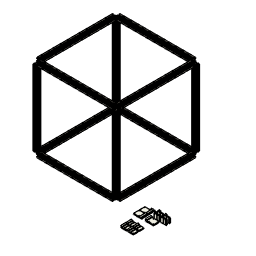
알루미늄 프로파일 20mm + 센서 케이스 v1+2+3 (Autodesk Fusion 360 design; units mm, degrees)
part number: 2025-07-09-12-54-32-083
Autodesk Fusion 360 part; units mm, degrees
note: some values were not read from the file. Set by a fixed rule: which sketch regions a step uses.
sketch "스케치1" plane through (0, 0, 0) normal (0, 0, 1) x (1, 0, 0)
  line L0 (20, 0) -> (17, 0)
  line L1 (20, 3) -> (20, 0)
  circle A0 centre (17, 3) radius 2
  circle A1 centre (17, 17) radius 2
  circle A2 centre (3, 17) radius 2
  circle A3 centre (3, 3) radius 2
  line L2 (12.65, 0) -> (12.65, 1.5)
  line L3 (12.65, 1.5) -> (14.15, 1.5)
  line L4 (14.15, 1.5) -> (14.15, 5.132)
  line L5 (7.35, 0) -> (7.35, 1.5)
  line L6 (7.35, 1.5) -> (5.85, 1.5)
  line L7 (5.85, 1.5) -> (5.85, 5.132)
  arc A4 (14.15, 5.132) -> (5.85, 5.132) centre (10, 0) ccw
  line L8 (0, 0) -> (7.35, 0)
  line L9 (12.65, 0) -> (20, 0)
  line L10 (12.65, 20) -> (12.65, 18.5)
  line L11 (12.65, 18.5) -> (14.15, 18.5)
  line L12 (14.15, 18.5) -> (14.15, 14.868)
  arc A5 (14.15, 14.868) -> (5.85, 14.868) centre (10, 20) cw
  line L13 (5.85, 18.5) -> (5.85, 14.868)
  line L14 (7.35, 18.5) -> (5.85, 18.5)
  line L15 (7.35, 20) -> (7.35, 18.5)
  line L16 (20, 12.65) -> (18.5, 12.65)
  line L17 (18.5, 12.65) -> (18.5, 14.15)
  line L18 (18.5, 14.15) -> (14.868, 14.15)
  arc A6 (14.868, 14.15) -> (14.868, 5.85) centre (20, 10) ccw
  line L19 (18.5, 5.85) -> (14.868, 5.85)
  line L20 (18.5, 7.35) -> (18.5, 5.85)
  line L21 (20, 7.35) -> (18.5, 7.35)
  line L22 (0, 7.35) -> (1.5, 7.35)
  line L23 (1.5, 7.35) -> (1.5, 5.85)
  line L24 (1.5, 5.85) -> (5.132, 5.85)
  arc A7 (5.132, 5.85) -> (5.132, 14.15) centre (0, 10) ccw
  line L25 (1.5, 14.15) -> (5.132, 14.15)
  line L26 (1.5, 12.65) -> (1.5, 14.15)
  line L27 (0, 12.65) -> (1.5, 12.65)
  line L28 (0, 20) -> (0, 12.65)
  line L29 (0, 7.35) -> (0, 0)
  line L30 (20, 0) -> (20, 7.35)
  line L31 (20, 12.65) -> (20, 20)
  line L32 (20, 20) -> (12.65, 20)
  line L33 (7.35, 20) -> (0, 20)
  line L34 (20, 12.65) -> (20, 7.35)
  dimension "d1" = 20
  dimension "d2" = 20
  dimension "d3" = 3
  dimension "d4" = 3
  dimension "d5" = 4
  dimension "d6" = 4
  dimension "d7" = 4
  dimension "d8" = 4
  dimension "d10" = 1.5
  dimension "d11" = 1.5
  dimension "d14" = 1.5
  dimension "d15" = 1.5
  dimension "d16" = 1.5
  dimension "d17" = 1.5
  dimension "d18" = 1.5
  dimension "d19" = 1.5
  dimension "d20" = 1.5
  dimension "d21" = 1.5
  dimension "d22" = 1.5
  dimension "d23" = 1.5
  dimension "d24" = 1.5
  dimension "d25" = 1.5
  dimension "d26" = 1.5
  dimension "d27" = 1.5
  constraint horizontal L8
  constraint vertical L30
  constraint horizontal L32
  constraint vertical L28
  constraint coincident L8.start L29.end
  constraint horizontal L0
  constraint vertical L1
  constraint perpendicular L2 L3
  constraint perpendicular L3 L4
  constraint perpendicular L5 L8
  constraint perpendicular L5 L6
  constraint perpendicular L6 L7
  constraint collinear L8 L9
  constraint perpendicular L10 L11
  constraint perpendicular L11 L12
  constraint perpendicular L14 L15
  constraint perpendicular L13 L14
  constraint perpendicular L16 L17
  constraint perpendicular L17 L18
  constraint perpendicular L20 L21
  constraint perpendicular L19 L20
  constraint perpendicular L22 L23
  constraint perpendicular L23 L24
  constraint perpendicular L26 L27
  constraint perpendicular L25 L26
  constraint collinear L28 L29
  constraint coincident A7.centre L28
  constraint collinear L30 L31
  constraint coincident A6.centre L30
  constraint collinear L32 L33
  constraint coincident A5.centre L32
  constraint perpendicular L21 L34
  measures "d1" distance of L8.start L0.start
  measures "d2" distance of L8.start L28.start
  measures "d3" distance of L0.start L0.end
  measures "d4" distance of L0.start L1.start
  measures "d5" diameter of A0
  measures "d6" diameter of A1
  measures "d7" diameter of A2
  measures "d8" diameter of A3
  measures "d10" distance of L2.start L2.end
  measures "d11" distance of L2.end L3.end
  measures "d14" distance of L5.start L5.end
  measures "d15" distance of L5.end L6.end
  measures "d16" distance of L10.start L10.end
  measures "d17" distance of L10.end L11.end
  measures "d18" distance of L14.start L15.start
  measures "d19" distance of L14.start L13.start
  measures "d20" distance of L16.start L16.end
  measures "d21" distance of L16.end L17.end
  measures "d22" distance of L20.start L21.start
  measures "d23" distance of L20.start L19.start
  measures "d24" distance of L22.start L22.end
  measures "d25" distance of L22.end L23.end
  measures "d26" distance of L26.start L27.start
  measures "d27" distance of L26.start L25.start
extrude "돌출1" add sketch "스케치1" along normal blind 400 contours L0 L1 L2 L3 L4 L5 L6 L7 A4 L8 L9 L10 L11 L12 A5 L13 L14 L15 L16 L17 L18 A6 L19 L20 L21 L22 L23 L24 A7 L25 L26 L27 L28 L29 L30 L31 L32 L33 | A0 | A1 | A2 | A3 makes body 1
move_body "이동1" bodies 1 to x (1, 0, 0) y (0, 0, -1) z (0, 1, 0) at (0, 0, 20)
move_body "이동2" bodies 1 to x (1, 0, 0) y (0, 1, 0) z (0, 0, 1) at (0, 20, 0)
move_body "이동3" bodies 1 to x (1, 0, 0) y (0, 1, 0) z (0, 0, 1) at (0, 5, 0)
extrude "돌출2" add sketch "스케치1" along normal blind 400 separate body contours L0 L1 L2 L3 L4 L5 L6 L7 A4 L8 L9 L10 L11 L12 A5 L13 L14 L15 L16 L17 L18 A6 L19 L20 L21 L22 L23 L24 A7 L25 L26 L27 L28 L29 L30 L31 L32 L33 makes body 2
move_body "이동4" bodies 2 to x (1, 0, 0) y (0, 1, 0) z (0, 0, 1) at (0, 0, 20)
move_body "이동5" bodies 1 to x (1, 0, 0) y (0, 1, 0) z (0, 0, 1) at (0, -5, 0)
copy_body "CopyPasteBodies1" bodies 1 makes body 3
move_body "이동6" bodies 3 to x (1, 0, 0) y (0, 1, 0) z (0, 0, 1) at (0, 0, 420)
copy_body "CopyPasteBodies2" bodies 2 makes body 4
move_body "이동7" bodies 4 to x (1, 0, 0) y (0, 1, 0) z (0, 0, 1) at (0, 420, 0)
extrude "돌출3" add sketch "스케치1" against normal blind 400 separate body contours L0 L1 L2 L3 L4 L5 L6 L7 A4 L8 L9 L10 L11 L12 A5 L13 L14 L15 L16 L17 L18 A6 L19 L20 L21 L22 L23 L24 A7 L25 L26 L27 L28 L29 L30 L31 L32 L33 makes body 5
move_body "이동8" bodies 5 to x (0, 0, 1) y (0, 1, 0) z (-1, 0, 0) at (-400, 0, 0)
copy_body "CopyPasteBodies3" bodies 5 makes body 6
move_body "이동9" bodies 6 to x (1, 0, 0) y (0, 1, 0) z (0, 0, 1) at (0, 420, 0)
copy_body "CopyPasteBodies4" bodies 5 makes body 7
move_body "이동10" bodies 7 to x (1, 0, 0) y (0, 1, 0) z (0, 0, 1) at (0, 0, 420)
copy_body "CopyPasteBodies5" bodies 6 makes body 8
move_body "이동11" bodies 8 to x (1, 0, 0) y (0, 1, 0) z (0, 0, 1) at (0, 0, 420)
copy_body "CopyPasteBodies6" bodies 2 makes body 9
move_body "이동12" bodies 9 to x (1, 0, 0) y (0, 1, 0) z (0, 0, 1) at (-420, 0, 0)
copy_body "CopyPasteBodies7" bodies 9 makes body 10
move_body "이동13" bodies 10 to x (1, 0, 0) y (0, 1, 0) z (0, 0, 1) at (0, 420, 0)
copy_body "CopyPasteBodies8" bodies 1 makes body 11
move_body "이동14" bodies 11 to x (1, 0, 0) y (0, 1, 0) z (0, 0, 1) at (-420, 0, 0)
copy_body "CopyPasteBodies9" bodies 11 makes body 12
move_body "이동15" bodies 12 to x (1, 0, 0) y (0, 1, 0) z (0, 0, 1) at (0, 0, 420)
extrude "돌출4" add sketch "스케치1" along normal blind 36 separate body contours L16 L17 L18 A6 L19 L20 L21 L34 makes body 13
move_body "이동16" bodies 13 to x (1, 0, 0) y (0, 1, 0) z (0, 0, 1) at (20, 0, 0)
move_body "이동17" bodies 13 to x (1, 0, 0) y (0, 0, 1) z (0, -1, 0) at (0, 5.85, -5.85)
move_body "이동18" bodies 13 to x (1, 0, 0) y (0, 1, 0) z (0, 0, 1) at (-20, 0, 6)
sketch "스케치9" plane through (0, -30.15, 0) normal (0, -1, 0) x (1, 0, 0)
  line L0 (18.5, 12.8) -> (18.5, 14.3)
  line L1 (18.5, 14.3) -> (14.868, 14.3)
  arc A0 (14.868, 14.3) -> (14.868, 6) centre (20, 10.15) ccw
  line L2 (14.868, 6) -> (18.5, 6)
  line L3 (18.5, 6) -> (18.5, 7.5)
  line L4 (18.5, 7.5) -> (20, 7.5)
  line L5 (20, 7.5) -> (20, 12.8)
  line L6 (20, 12.8) -> (18.5, 12.8)
  line L7 (20, 20) -> (15, 20)
  line L8 (15, 20) -> (15, 0)
  line L9 (15, 0) -> (20, 0)
  line L10 (20, 0) -> (20, 20)
  constraint horizontal L7
  constraint vertical L8
  constraint horizontal L9
  constraint vertical L10
extrude "돌출5" add sketch "스케치9" along normal blind 5 bodies 13
sketch "스케치10" plane through (20, 0, 0) normal (1, 0, 0) x (0, 1, 0)
  line L0 (5.85, 7.5) -> (5.85, 12.8)
  line L1 (5.85, 12.8) -> (-30.15, 12.8)
  line L2 (-30.15, 12.8) -> (-30.15, 20)
  line L3 (-30.15, 20) -> (-35.15, 20)
  line L4 (-35.15, 20) -> (-35.15, 0)
  line L5 (-35.15, 0) -> (-30.15, 0)
  line L6 (-30.15, 0) -> (-30.15, 7.5)
  line L7 (-30.15, 7.5) -> (5.85, 7.5)
  line L8 (-30.15, 7.5) -> (5.85, 7.5)
  line L9 (5.85, 7.5) -> (5.85, 49.5)
  line L10 (5.85, 49.5) -> (-30.15, 49.5)
  line L11 (-30.15, 49.5) -> (-30.15, 7.5)
  dimension "d38" = 42
  constraint horizontal L8
  constraint vertical L9
  constraint horizontal L10
  constraint vertical L11
  constraint coincident L6.end L7.start
  measures "d38" distance of L6.end L10.end
extrude "돌출6" add sketch "스케치10" along normal blind 5 contours L0 L1 L7 L8 L9 L11 | L1 L2 L9 L10 L11 bodies 13
extrude "돌출7" cut 1 faces at (23.3333, 5.85, 23.2667) along direction (0, -1, 0) blind 6.6 on bodies 13 bodies 13
sketch "스케치12" plane through (20, 0, 0) normal (-1, 0, 0) x (0, -1, 0)
  line L0 (0.75, 49.5) -> (0.75, 12.8)
  line L1 (0.75, 12.8) -> (30.15, 12.8)
  line L2 (30.15, 12.8) -> (30.15, 20)
  line L3 (30.15, 20) -> (30.15, 49.5)
  line L4 (30.15, 49.5) -> (0.75, 49.5)
  line L5 (30.15, 20) -> (0.75, 20)
  line L6 (30.15, 20) -> (26.85, 20)
  line L7 (26.85, 20) -> (26.85, 23.3)
  circle A0 centre (26.85, 23.3) radius 1.65
  line L8 (0.75, 20) -> (4.05, 20)
  line L9 (4.05, 20) -> (4.05, 21)
  line L10 (4.05, 20) -> (4.05, 23.3)
  line L11 (0.75, 49.5) -> (4.05, 49.5)
  line L12 (4.05, 49.5) -> (4.05, 46.2)
  line L13 (30.15, 49.5) -> (26.85, 49.5)
  line L14 (26.85, 49.5) -> (26.85, 46.2)
  circle A1 centre (4.05, 23.3) radius 1.65
  circle A2 centre (4.05, 46.2) radius 1.65
  circle A3 centre (26.85, 46.2) radius 1.65
  dimension "d46" = 3.3
  dimension "d47" = 3.3
  dimension "d48" = 3.3
  dimension "d49" = 3.3
  dimension "d50" = 3.3
  dimension "d51" = 3.3
  dimension "d52" = 3.3
  dimension "d53" = 3.3
  dimension "d54" = 3.3
  dimension "d55" = 3.3
  dimension "d56" = 3.3
  dimension "d57" = 3.3
  constraint coincident L2.end L3.start
  constraint coincident L0 L5.end
  constraint perpendicular L0 L5
  constraint perpendicular L2 L6
  constraint perpendicular L6 L7
  constraint coincident L7.end A0.centre
  constraint perpendicular L0 L8
  constraint perpendicular L5 L9
  constraint perpendicular L5 L10
  constraint coincident L0.start L4.end
  constraint perpendicular L0 L11
  constraint perpendicular L11 L12
  constraint coincident L3.end L4.start
  constraint perpendicular L3 L13
  constraint perpendicular L13 L14
  constraint coincident L10.end A1.centre
  constraint coincident L12.end A2.centre
  constraint coincident L14.end A3.centre
  measures "d46" distance of L2.end L6.end
  measures "d47" distance of L6.end L7.end
  measures "d48" diameter of A0
  measures "d49" distance of L5.end L8.end
  measures "d50" distance of L8.end L10.end
  measures "d51" distance of L0.start L11.end
  measures "d52" distance of L11.end L12.end
  measures "d53" distance of L3.end L13.end
  measures "d54" distance of L13.end L14.end
  measures "d55" diameter of A1
  measures "d56" diameter of A2
  measures "d57" diameter of A3
extrude "돌출8" cut sketch "스케치12" against normal blind 5 contours A0 | A1 | A2 | A3 bodies 13
mirror "미러1" about plane through (0, 0, 0) normal (1, 0, 0) of bodies 13 makes body 14
move_body "이동22" bodies 13 14 to x (1, 0, 0) y (0, 1, 0) z (0, 0, 1) at (180, 0, 0)
mirror "미러2" about plane through (0, 0, 0) normal (0, 1, 0) of bodies 13 makes body 15
mirror "미러3" about plane through (0, 0, 0) normal (0, 1, 0) of bodies 14 makes body 16
move_body "이동23" bodies 14 to x (0, 0, 1) y (0, 1, 0) z (-1, 0, 0) at (191.15, 0, -128.85)
move_body "이동24" bodies 16 to x (0, 0, 1) y (0, 1, 0) z (-1, 0, 0) at (191.15, 0, -128.85)
move_body "이동25" bodies 13 to x (0, 0, -1) y (0, 1, 0) z (1, 0, 0) at (153, 0, 252)
move_body "이동26" bodies 15 to x (0, 0, -1) y (0, 1, 0) z (1, 0, 0) at (153, 0, 252)
move_body "이동27" bodies 15 to x (1, 0, 0) y (0, 1, 0) z (0, 0, 1) at (45, 0, -20)
move_body "이동28" bodies 13 to x (1, 0, 0) y (0, 1, 0) z (0, 0, 1) at (45, 0, -20)
extrude "돌출9" cut 1 faces at (202.5, -35.15, 33.6667) along direction (0, 1, 0) blind 5 on bodies 13 bodies 13
sketch "스케치13" plane through (0, 0, 0) normal (0, 1, 0) x (1, 0, 0)
sketch "스케치14" plane through (0, 0, 32) normal (0, 0, 1) x (-1, 0, 0)
  circle A0 centre (-244.2, -26.85) radius 1.65
  circle A1 centre (-221.3, -4.05) radius 1.65
  circle A2 centre (-244.2, -4.05) radius 1.65
  circle A3 centre (-221.3, -26.85) radius 1.65
  line L0 (-210.8, -0.75) -> (-247.5, -0.75)
  line L1 (-247.5, -0.75) -> (-247.5, -30.15)
  line L2 (-247.5, -30.15) -> (-218, -30.15)
  line L3 (-218, -30.15) -> (-210.8, -30.15)
  line L4 (-210.8, -30.15) -> (-210.8, -0.75)
extrude "돌출10" add sketch "스케치14" against normal blind 5 contours A0 | A1 | A2 | A3 bodies 15
sketch "스케치15" plane through (0, 0, 32) normal (0, 0, 1) x (-1, 0, 0)
  line L0 (-210.8, -0.75) -> (-247.5, -0.75)
  line L1 (-247.5, -0.75) -> (-247.5, -30.15)
  line L2 (-247.5, -30.15) -> (-218, -30.15)
  line L3 (-218, -30.15) -> (-210.8, -30.15)
  line L4 (-210.8, -30.15) -> (-210.8, -0.75)
  line L5 (-218, -30.15) -> (-235.78, -30.15)
  line L6 (-235.78, -30.15) -> (-235.78, -0.75)
  line L7 (-235.78, -0.75) -> (-218, -0.75)
  line L8 (-218, -0.75) -> (-218, -30.15)
  dimension "d70" = 17.78
  constraint horizontal L5
  constraint vertical L6
  constraint horizontal L7
  constraint vertical L8
  constraint coincident L0 L6.end
  constraint coincident L2.end L3.start
  measures "d70" distance of L2.end L5.end
extrude "돌출11" cut sketch "스케치15" against normal blind 5 contours L0 L1 L2 L6 bodies 15
extrude "돌출12" cut 1 faces at (217.36, 0.75, 28.6667) along direction (0, 1, 0) blind 4 on bodies 15 bodies 15
sketch "스케치17" plane through (0, 0, 32) normal (0, 0, 1) x (-1, 0, 0)
sketch "스케치18" plane through (0, 0, 32) normal (0, 0, 1) x (-1, 0, 0)
  line L0 (-210.8, -4.75) -> (-235.78, -4.75)
  line L1 (-235.78, -4.75) -> (-235.78, -30.15)
  line L2 (-235.78, -30.15) -> (-218, -30.15)
  line L3 (-218, -30.15) -> (-210.8, -30.15)
  line L4 (-210.8, -30.15) -> (-210.8, -4.75)
  line L5 (-218, -30.15) -> (-218, -4.75)
  line L6 (-218, -30.15) -> (-220.54, -30.15)
  line L7 (-220.54, -30.15) -> (-220.54, -27.61)
  line L8 (-220.54, -27.61) -> (-218, -27.61)
  line L9 (-218, -27.61) -> (-218, -30.15)
  circle A0 centre (-220.54, -27.61) radius 1.27
  line L10 (-235.78, -30.15) -> (-233.24, -30.15)
  line L11 (-233.24, -30.15) -> (-233.24, -27.61)
  line L12 (-233.24, -27.61) -> (-235.78, -27.61)
  line L13 (-235.78, -27.61) -> (-235.78, -30.15)
  circle A1 centre (-233.24, -27.61) radius 1.27
  line L14 (-218, -4.75) -> (-220.54, -4.75)
  line L15 (-220.54, -4.75) -> (-220.54, -7.29)
  line L16 (-220.54, -7.29) -> (-218, -7.29)
  line L17 (-218, -7.29) -> (-218, -4.75)
  line L18 (-235.78, -4.75) -> (-233.24, -4.75)
  line L19 (-233.24, -4.75) -> (-233.24, -7.29)
  line L20 (-233.24, -7.29) -> (-235.78, -7.29)
  line L21 (-235.78, -7.29) -> (-235.78, -4.75)
  circle A2 centre (-220.54, -7.29) radius 1.27
  circle A3 centre (-233.24, -7.29) radius 1.27
  dimension "d75" = 2.54
  dimension "d76" = 2.54
  dimension "d77" = 2.54
  dimension "d78" = 2.54
  dimension "d79" = 2.54
  dimension "d80" = 2.54
  dimension "d81" = 2.54
  dimension "d82" = 2.54
  dimension "d83" = 2.54
  dimension "d84" = 2.54
  dimension "d85" = 2.54
  dimension "d86" = 2.54
  constraint coincident L2.end L3.start
  constraint coincident L0 L5.end
  constraint perpendicular L0 L5
  constraint horizontal L6
  constraint vertical L7
  constraint horizontal L8
  constraint vertical L9
  constraint coincident L7.end L8.start
  constraint horizontal L10
  constraint vertical L11
  constraint horizontal L12
  constraint vertical L13
  constraint coincident L1.end L2.start
  constraint coincident L11.end L12.start
  constraint horizontal L14
  constraint vertical L15
  constraint horizontal L16
  constraint vertical L17
  constraint horizontal L18
  constraint vertical L19
  constraint horizontal L20
  constraint vertical L21
  constraint coincident L0.end L1.start
  constraint coincident L15.end L16.start
  constraint coincident L19.end L20.start
  measures "d75" distance of L2.end L6.end
  measures "d76" distance of L2.end L8.end
  measures "d77" diameter of A0
  measures "d78" distance of L1.end L10.end
  measures "d79" distance of L1.end L12.end
  measures "d80" diameter of A1
  measures "d81" distance of L5.end L14.end
  measures "d82" distance of L5.end L16.end
  measures "d83" distance of L0.end L18.end
  measures "d84" distance of L0.end L20.end
  measures "d85" diameter of A2
  measures "d86" diameter of A3
extrude "돌출13" cut sketch "스케치18" against normal blind 5 contours L15 L16 A2 | L15 L16 A2 | L19 L20 A3 | L19 L20 A3 | L7 L8 A0 | L7 L8 A0 | L11 L12 A1 | L11 L12 A1 bodies 15
extrude "돌출14" cut 1 faces at (202.5, 35.15, 33.6667) along direction (0, -1, 0) blind 5 on bodies 15 bodies 15
sketch "스케치19" plane through (0, 0, 32) normal (0, 0, 1) x (-1, 0, 0)
  circle A0 centre (-233.24, -27.61) radius 1.27
  circle A1 centre (-233.24, -7.29) radius 1.27
  circle A2 centre (-220.54, -27.61) radius 1.27
  circle A3 centre (-220.54, -7.29) radius 1.27
  line L0 (-210.8, -4.75) -> (-235.78, -4.75)
  line L1 (-235.78, -4.75) -> (-235.78, -30.15)
  line L2 (-235.78, -30.15) -> (-210.8, -30.15)
  line L3 (-210.8, -30.15) -> (-210.8, -4.75)
  line L4 (-220.54, -27.61) -> (-221.175, -27.61)
  line L5 (-221.175, -27.61) -> (-219.905, -27.61)
  line L6 (-219.905, -27.61) -> (-219.905, -7.29)
  line L7 (-219.905, -7.29) -> (-221.175, -7.29)
  line L8 (-221.175, -7.29) -> (-221.175, -27.61)
  line L9 (-233.24, -27.61) -> (-232.605, -27.61)
  line L10 (-232.605, -27.61) -> (-233.875, -27.61)
  line L11 (-233.875, -27.61) -> (-233.875, -7.29)
  line L12 (-233.875, -7.29) -> (-232.605, -7.29)
  line L13 (-232.605, -7.29) -> (-232.605, -27.61)
  dimension "d91" = 0.635
  dimension "d92" = 1.27
  dimension "d93" = 20.32
  dimension "d94" = 0.635
  dimension "d95" = 1.27
  dimension "d96" = 20.32
  constraint coincident A2.centre L4.start
  constraint horizontal L4
  constraint horizontal L5
  constraint vertical L6
  constraint horizontal L7
  constraint vertical L8
  constraint coincident A0.centre L9.start
  constraint parallel L2 L9
  constraint horizontal L10
  constraint vertical L11
  constraint horizontal L12
  constraint vertical L13
  measures "d91" distance of A2.centre L4.end
  measures "d92" distance of L4.end L5.end
  measures "d93" distance of L4.end L7.end
  measures "d94" distance of A0.centre L9.end
  measures "d95" distance of L9.end L10.end
  measures "d96" distance of L9.end L12.end
extrude "돌출15" cut sketch "스케치19" against normal blind 5 contours A0 A1 L11 L13 | A2 A3 L6 L8 bodies 15
copy_body "CopyPasteBodies11" bodies 15 makes body 17
move_body "이동29" bodies 15 17 to x (1, 0, 0) y (0, 0, -1) z (0, 1, 0) at (0, -12.05, 46.95)
copy_body "CopyPasteBodies12" bodies 15 makes body 18
move_body "이동30" bodies 18 to x (1, 0, 0) y (0, 1, 0) z (0, 0, 1) at (34, 0, 0)
copy_body "CopyPasteBodies14" bodies 18 15 makes body 19 makes body 20
move_body "이동32" bodies 19 20 to x (1, 0, 0) y (0, 1, 0) z (0, 0, 1) at (0, 17, 0)
sketch "스케치20" plane through (0, 19.95, 0) normal (0, 1, 0) x (-1, 0, 0)
  line L0 (-233.875, 20.4399) -> (-233.875, 38.5601)
  arc A0 (-232.605, 38.5601) -> (-233.875, 38.5601) centre (-233.24, 39.66) ccw
  line L1 (-232.605, 38.5601) -> (-232.605, 20.4399)
  arc A1 (-233.875, 20.4399) -> (-232.605, 20.4399) centre (-233.24, 19.34) ccw
  line L2 (-219.905, 38.5601) -> (-219.905, 20.4399)
  arc A2 (-221.175, 20.4399) -> (-219.905, 20.4399) centre (-220.54, 19.34) ccw
  line L3 (-221.175, 20.4399) -> (-221.175, 38.5601)
  arc A3 (-219.905, 38.5601) -> (-221.175, 38.5601) centre (-220.54, 39.66) ccw
  line L4 (-210.8, 42.2) -> (-235.78, 42.2)
  line L5 (-235.78, 42.2) -> (-235.78, 16.8)
  line L6 (-235.78, 16.8) -> (-210.8, 16.8)
  line L7 (-210.8, 16.8) -> (-210.8, 42.2)
  line L8 (-221.175, 38.5601) -> (-219.905, 38.5601)
  line L9 (-219.905, 38.5601) -> (-219.905, 20.4399)
  line L10 (-219.905, 20.4399) -> (-221.175, 20.4399)
  line L11 (-221.175, 20.4399) -> (-221.175, 38.5601)
  line L12 (-220.54, 29.5) -> (-220.54, 37.5)
  line L13 (-220.54, 37.5) -> (-219.24, 37.5)
  line L14 (-219.24, 37.5) -> (-221.84, 37.5)
  line L15 (-221.84, 37.5) -> (-221.84, 21.5)
  line L16 (-221.84, 21.5) -> (-219.24, 21.5)
  line L17 (-219.24, 21.5) -> (-219.24, 37.5)
  circle A4 centre (-220.54, 39.66) radius 1.27
  circle A5 centre (-220.54, 19.34) radius 1.27
  circle A6 centre (-233.24, 19.34) radius 1.27
  circle A7 centre (-233.24, 39.66) radius 1.27
  line L18 (-220.54, 29.5) -> (-232.605, 29.5)
  line L19 (-232.605, 29.5) -> (-231.94, 29.5)
  line L20 (-231.94, 29.5) -> (-231.94, 37.5)
  line L21 (-231.94, 37.5) -> (-234.54, 37.5)
  line L22 (-234.54, 37.5) -> (-234.54, 21.5)
  line L23 (-234.54, 21.5) -> (-231.94, 21.5)
  line L24 (-231.94, 21.5) -> (-231.94, 37.5)
  dimension "d99" = 8
  dimension "d100" = 1.3
  dimension "d101" = 2.6
  dimension "d102" = 16
  dimension "d103" = 0.665
  dimension "d104" = 8
  dimension "d105" = 2.6
  dimension "d106" = 16
  constraint horizontal L8
  constraint vertical L9
  constraint horizontal L10
  constraint vertical L11
  constraint coincident L2.end A2.end
  constraint coincident L3.end A3.end
  constraint parallel L2 L12
  constraint perpendicular L2 L13
  constraint horizontal L14
  constraint vertical L15
  constraint horizontal L16
  constraint vertical L17
  constraint concentric A3 A4
  constraint concentric A2 A5
  constraint concentric A1 A6
  constraint concentric A0 A7
  constraint midpoint L1 L18.end
  constraint perpendicular L1 L19
  constraint perpendicular L19 L20
  constraint horizontal L21
  constraint vertical L22
  constraint horizontal L23
  constraint vertical L24
  measures "d99" distance of L12.start L12.end
  measures "d100" distance of L12.end L13.end
  measures "d101" distance of L13.end L14.end
  measures "d102" distance of L13.end L16.end
  measures "d103" distance of L18.end L19.end
  measures "d104" distance of L19.end L20.end
  measures "d105" distance of L20.end L21.end
  measures "d106" distance of L20.end L23.end
extrude "돌출16" add sketch "스케치20" against normal blind 5 contours L0 L1 A6 L23 | L0 L1 A7 L21 | L2 L3 L9 L11 L13 L14 A4 | L2 L3 L9 L11 L16 A5 bodies 15
extrude "돌출17" cut sketch "스케치20" against normal blind 5 contours L0 L21 L22 L23 | L1 L18 L19 L23 L24 | L1 L18 L19 L20 L21 L24 | L2 L9 L13 L14 L16 L17 | L3 L11 L14 L15 L18 | L3 L11 L15 L16 L18 bodies 15
sketch "스케치21" plane through (0, 19.95, 0) normal (0, 1, 0) x (-1, 0, 0)
extrude "돌출18" add sketch "스케치20" against normal blind 5 contours L0 L21 L22 L23 | L0 L1 L21 L23 | L1 L18 L19 L23 L24 | L1 L18 L19 L20 L21 L24 bodies 15
move_body "이동33" bodies 15 to x (1, 0, 0) y (0, 0, 1) z (0, -1, 0) at (0, 46.95, 12.05)
copy_body "CopyPasteBodies15" bodies 15 makes body 21
move_body "이동34" bodies 21 to x (1, 0, 0) y (0, 1, 0) z (0, 0, 1) at (0, -30, 0)
copy_body "CopyPasteBodies16" bodies 21 15 makes body 22 makes body 23
move_body "이동35" bodies 22 23 to x (1, 0, 0) y (0, 1, 0) z (0, 0, 1) at (-35, 0, 0)
move_body "Move36" bodies 21 22 15 23 to x (1, 0, 0) y (0, 1, 0) z (0, 0, 1) at (0, -100, 0)
equation "d38 = 12.5 mm + 29.5 mm"
equation "d44 = 29.4 mm - 36 mm"
